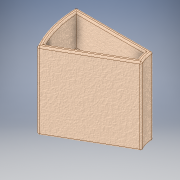
# Autodesk Inventor part: angular30
Saved by Autodesk Inventor 2019 (Build 230136000, 136)
## iProperties
Created: 2019-02-27
Part Number: angular30
Material: Concrete
Document SubType Name: Modeling
Designer: gaincarlo
Density: 2.40731 g/cm^3
Appearance: Exterior - Beige
Author: gaincarlo
Autodesk Inventor part; units mm, degrees
ref_plane "YZ Plane" through (0, 0, 0) normal (1, 0, 0) x (0, 1, 0)
ref_plane "XZ Plane" through (0, 0, 0) normal (0, 1, 0) x (-1, 0, 0)
ref_plane "XY Plane" through (0, 0, 0) normal (0, 0, 1) x (1, 0, 0)
sketch "Sketch1" plane through (0, 0, 0) normal (0, 1, 0) x (-1, 0, 0)
  line L0 (0, 0) -> (500, 0)
  arc A0 (500, 0) -> (406.3518, 349.5) centre (-199, 0) ccw
  arc A1 (0, 0) -> (-26.6609, 99.5) centre (-199, 0) ccw
  line L1 (-26.6609, 99.5) -> (406.3518, 349.5)
  line L2 (-343.4013, 0) -> (667.4075, 0) projected
  dimension "d1" = 500
  dimension "d2" = 30
  constraints: 4 end point, 4 point on circle, 3 point on line, 2 centre point, 1 coincident, 1 horizontal
  measures "d1" distance of L0.start L0.end
  measures "d2" angle of L0 L1
extrude "Extrusion1" add sketch "Sketch1" along normal blind 500
sketch "Sketch2" plane through (0, 500, 0) normal (0, 1, 0) x (1, 0, 0)
  arc A0 (0, 0) -> (26.6609, -99.5) centre (199, 0) ccw projected
  line L0 (26.6609, -99.5) -> (-406.3518, -349.5) projected
  arc A1 (-500, 0) -> (-406.3518, -349.5) centre (199, 0) ccw projected
  line L1 (-500, 0) -> (0, 0) projected
  line L2 (-394.7882, -308.1827) -> (-12.6107, -87.5325)
  arc A2 (-28.0264, -30) -> (-12.6107, -87.5325) centre (199, 0) ccw
  line L3 (-28.0264, -30) -> (-469.327, -30)
  arc A3 (-469.327, -30) -> (-394.7882, -308.1827) centre (199, 0) ccw
  dimension "d5" = 30
  constraints: 4 end point, 4 point on circle, 2 centre point, 3 other
  measures "d5" radial gap between concentric circles of A1 A3
extrude "Extrusion2" cut sketch "Sketch2" against normal blind 200 contours A3 L3 A2 L2
fillet "Fillet1" radius 10 16 edges at (-189.8454, 0, 224.5) (26.6609, 250, 99.5) (-189.8454, 500, 224.5) (-406.3518, 250, 349.5) (6.7808, 0, 51.505) (0, 250, 0) (6.7808, 500, 51.505) (-250, 0, 0) (-500, 250, 0) (-250, 500, 0) (-476.1822, 0, 180.9145) (-476.1822, 500, 180.9145) (-22.197, 500, 59.2696) (-203.6994, 500, 197.8576) (-447.2044, 500, 173.1499) (-248.6767, 500, 30)
body "Solid1"
